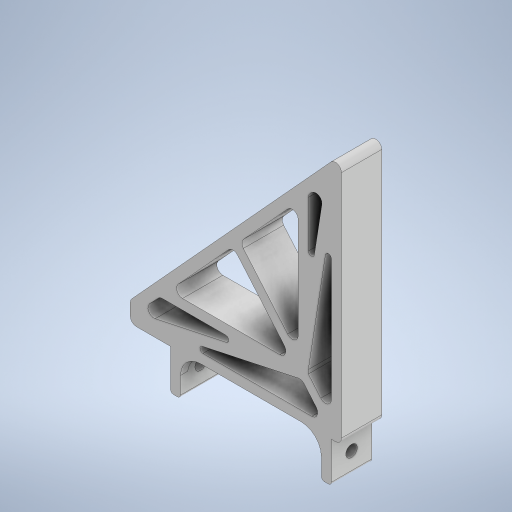
# Autodesk Inventor part: Controls Mid Support
Saved by Autodesk Inventor 2024.1 (Build 281209000, 209)
## iProperties
Created: 2023-10-28
Part Number: Controls Mid Support
Material: Generic
Document SubType Name: Modeling
Designer: david
Density: 1 g/cm^3
Appearance: Default
Author: david
Autodesk Inventor part; units mm, degrees
ref_plane "YZ Plane" through (0, 0, 0) normal (1, 0, 0) x (0, 1, 0)
ref_plane "XZ Plane" through (0, 0, 0) normal (0, 1, 0) x (-1, 0, 0)
ref_plane "XY Plane" through (0, 0, 0) normal (0, 0, 1) x (1, 0, 0)
sketch "Sketch1" plane through (0, 0, 0) normal (0, 0, 1) x (1, 0, 0)
  line L0 (0, 0) -> (0, 125)
  line L1 (0, 125) -> (-105, 10)
  line L2 (-105, 10) -> (-105, 0)
  line L3 (-105, 0) -> (0, 0)
  line L4 (-100, 8.0608) -> (-5, 112.1084)
  line L5 (-5, 112.1084) -> (-5, 5)
  line L6 (-5, 5) -> (-100, 5)
  line L7 (-100, 5) -> (-100, 8.0608)
  point P0 (-52.5, 62.5)
  point P1 (-52.5, 0)
  point P2 (0, 62.5)
  dimension "d0" = 10
  dimension "d1" = 105
  dimension "d2" = 125
  dimension "d3" = 5
  constraints: 16 end point, 2 midpoint, 2 parallel, 2 perpendicular, 1 horizontal alignment, 1 vertical, 1 vertical alignment, 3 other
  measures "d0" distance of L1.end L2.end
  measures "d1" distance of L2.end L0.start
  measures "d2" distance of L0.start L0.end
  measures "d3" distance between parallel lines of L0 L5
extrude "Extrusion1" add sketch "Sketch1" along normal blind 20
sketch "Sketch2" plane through (0, 0, 0) normal (0, 0, -1) x (-1, 0, 0)
  line L0 (5, 112.1084) -> (5, 5) projected
  line L1 (5, 8.8556) -> (50.4993, 62.2758)
  line L2 (100, 8.0608) -> (5, 112.1084) projected
  line L3 (5, 5) -> (100, 5) projected
  line L4 (8.2839, 5) -> (53.8973, 58.5542)
  line L5 (16.4791, 22.3331) -> (16.4791, 99.536)
  line L6 (21.4791, 94.0598) -> (21.4791, 28.2035)
  line L7 (24.1213, 23.5946) -> (85.817, 23.5946)
  line L8 (19.8627, 18.5946) -> (90.3822, 18.5946)
  line L9 (100, 5) -> (100, 8.0608) projected
  line L10 (100, 6.5304) -> (23.4466, 22.8023)
  line L11 (83.1512, 5) -> (19.7602, 18.4742)
  line L12 (8.1824, 108.6229) -> (21.0073, 27.6496)
  line L13 (5, 96.7537) -> (16.7388, 22.6379)
  point P0 (0, 0)
  point P1 (16.4791, 56.2397)
  point P2 (43.2425, 18.5946)
  point P3 (16.4791, 24.2774)
  dimension "d8" = 2.5
  dimension "d9" = 2.5
  dimension "d10" = 5
  dimension "d11" = 5
  dimension "d16" = 5
  dimension "d17" = 12
  dimension "d18" = 5
  dimension "d19" = 9
  constraints: 20 end point, 12 point on line, 5 parallel, 1 horizontal, 1 midpoint, 1 vertical, 8 other
  measures "d8" distance from line of L4 L0.end
  measures "d9" distance from line of L0.end L1
  measures "d10" distance between parallel lines of L6 L5
  measures "d11" distance between parallel lines of L8 L7
  measures "d16" distance between parallel lines of L11 L10
  measures "d17" angle of L3 L11
  measures "d18" distance between parallel lines of L13 L12
  measures "d19" angle of L0 L13
extrude "Extrusion2" add sketch "Sketch2" against normal blind 20 contours L2 L12 L5 L13 L0 | L1 L2 L4 L3 L0 | L13 L1 L5 | L5 L12 L1 L13 | L2 L6 L1 L12 L5 | L11 L4 L8 L10 L9 L3 | L4 L10 L8 | L2 L8 L10 L4 L7
fillet "Fillet1" radius 3 18 edges at (-90.3822, 18.5946, 10) (-53.8973, 58.5542, 10) (-85.817, 23.5946, 10) (-24.1213, 23.5946, 10) (-50.4993, 62.2758, 10) (-21.4791, 94.0598, 10) (-16.4791, 99.536, 10) (-21.4791, 28.2035, 10) (0, 0, 10) (-5, 8.8556, 10) (-8.2839, 5, 10) (-105, 0, 10) (-100, 8.0608, 10) (-105, 10, 10) (0, 125, 10) (-19.7602, 18.4742, 10) (-100, 6.5304, 10) (-8.1824, 108.6229, 10)
fillet "Fillet2" radius 1.5 4 edges at (-16.4791, 56.2397, 10) (-43.2425, 18.5946, 10) (-5, 96.7537, 10) (-83.1512, 5, 10)
sketch "Sketch5" plane through (0, 0, 20) normal (0, 0, 1) x (1, 0, 0)
  line L0 (-102, 0) -> (-3, 0) projected
  line L1 (-85, 0) -> (-85, -20)
  line L2 (-80, 0) -> (-80, -20)
  line L3 (-80, -20) -> (-85, -20)
  line L4 (-10, 0) -> (-10, -20)
  line L5 (-10, -20) -> (-5, -20)
  line L6 (-5, -20) -> (-5, 0)
  line L7 (-105, 8.8365) -> (-105, 3) projected
  point P0 (0, 0)
  dimension "d35" = 5
  dimension "d36" = 20
  dimension "d37" = 80
  dimension "d38" = 5
  dimension "d52" = 20
  constraints: 12 end point, 4 point on line, 3 perpendicular, 3 vertical, 1 horizontal alignment
  measures "d35" distance between parallel lines of L2 L1
  measures "d36" distance between parallel lines of L7 L1
  measures "d37" distance between parallel lines of L6 L1
  measures "d38" distance between parallel lines of L4 L6
  measures "d52" distance of L1.start L1.end
extrude "Extrusion3" add sketch "Sketch5" against normal up to surface (20 mm away)
fillet "Fillet3" radius 1.5 4 edges at (-80, -20, 10) (-85, -20, 10) (-10, -20, 10) (-5, -20, 10)
fillet "Fillet4" radius 10 2 edges at (-80, 0, 10) (-10, 0, 10)
sketch "Sketch6" plane through (-10, -18.5, 0) normal (-1, 0, 0) x (0, 0, 1)
  line L0 (0, -1.5) -> (20, -1.5) projected
  line L1 (0, 0) -> (0, 8.5) projected
  point P0 (0, 18.5)
  point P1 (10, 8.5)
  dimension "d50" = 10
  dimension "d51" = 10
  measures "d50" distance from line of point (10, 8.5) L0
  measures "d51" distance from line of L1 point (10, 8.5)
hole "Hole2" at (-10, -10, 10) direction (1, 0, 0) diameter 5.8 end through all clearance for "Flat Head Machine Screw" size "M5" standard "Ansi Metric M Profile"
sketch "Sketch7" plane through (-10, -18.5, 0) normal (-1, 0, 0) x (0, 0, 1)
  arc A0 (12.9, 8.5) -> (7.1, 8.5) centre (10, 8.5) ccw projected
  circle A1 centre (10, 8.5) radius 6.4
  arc A2 (7.1, 8.5) -> (12.9, 8.5) centre (10, 8.5) ccw projected
  point P0 (0, 18.5)
  dimension "d53" = 3.5
  constraints: 1 centre point, 1 coincident
  measures "d53" radial gap between concentric circles of A1 A2
extrude "Extrusion4" cut sketch "Sketch7" along normal blind 10 contours A2 A0 | A1
sketch "Sketch8" plane through (-80, -18.5, 20) normal (1, 0, 0) x (0, 0, -1)
  line L0 (20, 8.5) -> (20, 0) projected
  line L1 (0, -1.5) -> (20, -1.5) projected
  point P0 (20, 18.5)
  point P1 (10, 8.5)
  dimension "d63" = 10
  dimension "d64" = 10
  measures "d63" distance from line of L0 point (10, 8.5)
  measures "d64" distance from line of L1 point (10, 8.5)
hole "Hole3" at (-80, -10, 10) direction (-1, 0, 0) diameter 5.8 end through all clearance for "Flat Head Machine Screw" size "M5" standard "Ansi Metric M Profile"
sketch "Sketch9" plane through (-80, -18.5, 20) normal (1, 0, 0) x (0, 0, -1)
  line L0 (7.1, 8.5) -> (12.9, 8.5) projected
  circle A0 centre (10, 8.5) radius 6.4
  point P0 (20, 18.5)
  constraints: 1 centre point, 1 midpoint
extrude "Extrusion5" cut sketch "Sketch9" along normal blind 10
equation "\"d9\" = d8"
equation "\"d35\" = d38"
body "Solid1"
